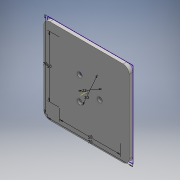
# Autodesk Inventor part: support_plateau_v3
Saved by Autodesk Inventor 2016 (Build 200138000, 138)
## iProperties
Created: 2018-02-19
Part Number: support_plateau_v3
Material: Generic
Document SubType Name: Modeling
Designer: mbouhier
Density: 1 g/cm^3
Appearance: Default
Author: mbouhier
Autodesk Inventor part; units mm, degrees
ref_plane "YZ Plane" through (0, 0, 0) normal (1, 0, 0) x (0, 1, 0)
ref_plane "XZ Plane" through (0, 0, 0) normal (0, 1, 0) x (-1, 0, 0)
ref_plane "XY Plane" through (0, 0, 0) normal (0, 0, 1) x (1, 0, 0)
sketch "Sketch1" plane through (0, 0, 0) normal (0, 1, 0) x (-1, 0, 0)
  line L0 (-35, 35) -> (35, 35)
  line L1 (35, 35) -> (35, -35)
  line L2 (35, -35) -> (-35, -35)
  line L3 (-35, -35) -> (-35, 35)
  line L4 (-35, 35) -> (35, -35) construction
  line L5 (35, 35) -> (-35, -35) construction
  line L6 (-25, 25) -> (25, 25)
  line L7 (25, 25) -> (25, -25)
  line L8 (25, -25) -> (-25, -25)
  line L9 (-25, -25) -> (-25, 25)
  line L10 (-25, 25) -> (25, -25) construction
  line L11 (25, 25) -> (-25, -25) construction
  circle A0 centre (0, 0) radius 15 construction
  circle A1 centre (0, 0) radius 11 construction
  point P0 (15, 0)
  dimension "d4" = 30
  dimension "d0" = 70
  dimension "d1" = 70
  dimension "d2" = 50
  dimension "d3" = 50
  dimension "d5" = 22
  constraints: 24 end point, 6 midpoint, 4 parallel, 2 coincident, 2 horizontal, 2 perpendicular, 1 centre point, 1 horizontal alignment, 2 other
  measures "d0" distance of L1.end L2.end
  measures "d1" distance of L0.end L1.end
  measures "d2" distance of L7.end L8.end
  measures "d3" distance of L6.end L7.end
  measures "d5" diameter of A1
extrude "Extrusion1" add sketch "Sketch1" along normal blind 3 contours L6 L7 L8 L9
extrude "Extrusion2" add sketch "Sketch1" against normal blind 3 contours L0 L1 L2 L3 | L6 L7 L8 L9
sketch "Sketch2" plane through (0, 3, 0) normal (0, 1, 0) x (1, 0, 0)
  circle A0 centre (0, 0) radius 11 construction
  circle A1 centre (0, 0) radius 15 construction
  point P0 (11, 0)
  constraints: 1 centre point, 1 horizontal alignment, 2 other
hole "Hole1" at (11, 3, 0) direction (0, -1, 0) diameter 4.1 end through all counterbore diameter 7.5 counterbore depth 4.2
pattern_circular "Circular Pattern1" count 3 over 360 about axis through (0, 3, 0) along (0, -1, 0) of "Hole1"
fillet "Fillet1" radius 5 8 edges at (35, -1.5, 35) (-35, -1.5, 35) (-35, -1.5, -35) (35, -1.5, -35) (25, 1.5, -25) (25, 1.5, 25) (-25, 1.5, 25) (-25, 1.5, -25)
sketch "Sketch3" plane through (0, -3, 0) normal (0, -1, 0) x (1, 0, 0)
  circle A0 centre (0, 0) radius 1
  dimension "d21" = 2
  constraints: 2 coincident, 1 centre point
  measures "d21" diameter of A0
extrude "Extrusion3" cut sketch "Sketch3" against normal blind 0.1
body "Solid1"
